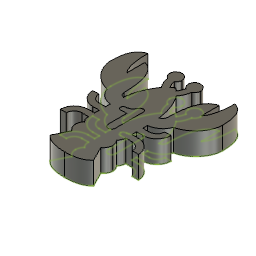
lobster-meeple-1 (Autodesk Fusion 360 design; units mm, degrees)
part number: 2026-09-20-14-42-37-938
Autodesk Fusion 360 part; units mm, degrees
sketch "Sketch4" plane through (0, 0, 0) normal (0, 0, 1) x (1, 0, 0)
  spline S0 degree 3 poles (20.1551, -11.6126) (23.0817, -10.9889) (25.2713, -8.149) (25.2713, -5.6734) knots 0 0 0 0 1 1 1 1
  spline S1 degree 2 poles (25.2713, -5.6734) (25.2713, -0.7748) (22.4721, -0.075) knots 0 0 0 1 1 1
  spline S2 degree 3 poles (22.4721, -0.075) (22.4721, -5.0901) (21.1273, -6.0667) (21.0725, -6.1398) knots 0 0 0 0 1 1 1 1
  line L0 (21.0725, -6.1398) -> (21.0725, -2.1744)
  spline S3 degree 3 poles (21.0725, -2.1744) (17.5735, -2.8742) (17.5735, -8.939) (17.5735, -10.3387) knots 0 0 0 0 1 1 1 1
  spline S4 degree 3 poles (17.5735, -10.3387) (17.5735, -10.8576) (17.1946, -11.2887) (16.6992, -11.3725) knots 0 0 0 0 1 1 1 1
  spline S5 degree 3 poles (16.6992, -11.3725) (16.295, -8.2827) (15.2588, -6.3478) (14.3388, -5.1927) knots 0 0 0 0 1 1 1 1
  spline S6 degree 3 poles (14.3388, -5.1927) (14.7426, -4.751) (15.2127, -3.9854) (15.3954, -2.7274) knots 0 0 0 0 1 1 1 1
  spline S7 degree 3 poles (15.3954, -2.7274) (15.8563, -2.4984) (16.1739, -2.0241) (16.1739, -1.4746) knots 0 0 0 0 1 1 1 1
  spline S8 degree 3 poles (16.1739, -1.4746) (16.1739, -0.7017) (15.5472, -0.075) (14.7743, -0.075) knots 0 0 0 0 1 1 1 1
  spline S9 degree 3 poles (14.7743, -0.075) (14.0013, -0.075) (13.3747, -0.7017) (13.3747, -1.4746) knots 0 0 0 0 1 1 1 1
  spline S10 degree 3 poles (13.3747, -1.4746) (13.3747, -1.9583) (13.6201, -2.3845) (13.9931, -2.636) knots 0 0 0 0 1 1 1 1
  spline S11 degree 3 poles (13.9931, -2.636) (13.859, -3.4351) (13.5844, -3.9119) (13.3647, -4.1785) knots 0 0 0 0 1 1 1 1
  spline S12 degree 2 poles (13.3647, -4.1785) (12.9526, -3.8299) (12.675, -3.6906) knots 0 0 0 1 1 1
  spline S13 degree 2 poles (12.675, -3.6906) (12.3973, -3.8299) (11.9853, -4.1785) knots 0 0 0 1 1 1
  spline S14 degree 3 poles (11.9853, -4.1785) (11.7655, -3.9119) (11.4909, -3.4351) (11.3568, -2.636) knots 0 0 0 0 1 1 1 1
  spline S15 degree 3 poles (11.3568, -2.636) (11.7298, -2.3845) (11.9753, -1.9582) (11.9753, -1.4746) knots 0 0 0 0 1 1 1 1
  spline S16 degree 3 poles (11.9753, -1.4746) (11.9753, -0.7017) (11.3486, -0.075) (10.5757, -0.075) knots 0 0 0 0 1 1 1 1
  spline S17 degree 3 poles (10.5757, -0.075) (9.8027, -0.075) (9.1761, -0.7017) (9.1761, -1.4746) knots 0 0 0 0 1 1 1 1
  spline S18 degree 3 poles (9.1761, -1.4746) (9.1761, -2.0242) (9.4936, -2.4984) (9.9545, -2.7274) knots 0 0 0 0 1 1 1 1
  spline S19 degree 3 poles (9.9545, -2.7274) (10.1372, -3.9854) (10.6074, -4.751) (11.0111, -5.1927) knots 0 0 0 0 1 1 1 1
  spline S20 degree 3 poles (11.0111, -5.1927) (10.0912, -6.3478) (9.055, -8.2827) (8.6508, -11.3725) knots 0 0 0 0 1 1 1 1
  spline S21 degree 3 poles (8.6508, -11.3725) (8.1553, -11.2887) (7.7765, -10.8576) (7.7765, -10.3387) knots 0 0 0 0 1 1 1 1
  spline S22 degree 3 poles (7.7765, -10.3387) (7.7765, -8.9391) (7.7765, -2.8742) (4.2775, -2.1744) knots 0 0 0 0 1 1 1 1
  line L1 (4.2775, -2.1744) -> (4.2775, -6.1398)
  spline S23 degree 3 poles (4.2775, -6.1398) (4.2226, -6.0667) (2.8779, -5.0901) (2.8779, -0.075) knots 0 0 0 0 1 1 1 1
  spline S24 degree 2 poles (2.8779, -0.075) (0.0787, -0.7748) (0.0787, -5.6734) knots 0 0 0 1 1 1
  spline S25 degree 3 poles (0.0787, -5.6734) (0.0787, -8.149) (2.2683, -10.989) (5.1949, -11.6126) knots 0 0 0 0 1 1 1 1
  spline S26 degree 3 poles (5.1949, -11.6126) (5.6849, -13.0051) (6.9538, -14.0331) (8.4764, -14.1709) knots 0 0 0 0 1 1 1 1
  spline S27 degree 3 poles (8.4764, -14.1709) (8.4764, -14.1765) (8.4763, -14.1819) (8.4763, -14.1875) knots 0 0 0 0 1 1 1 1
  line L2 (8.4763, -14.1875) -> (8.4763, -15.2372)
  line L3 (8.4763, -15.2372) -> (7.0067, -15.2372)
  spline S28 degree 3 poles (7.0067, -15.2372) (6.042, -15.2372) (5.2572, -14.4524) (5.2572, -13.4877) knots 0 0 0 0 1 1 1 1
  line L4 (5.2572, -13.4877) -> (3.8576, -13.4877)
  spline S29 degree 3 poles (3.8576, -13.4877) (3.8576, -15.2241) (5.2703, -16.6368) (7.0067, -16.6368) knots 0 0 0 0 1 1 1 1
  line L5 (7.0067, -16.6368) -> (8.4763, -16.6368)
  line L6 (8.4763, -16.6368) -> (8.4763, -17.6865)
  line L7 (8.4763, -17.6865) -> (7.0067, -17.6865)
  spline S30 degree 3 poles (7.0067, -17.6865) (5.2703, -17.6865) (3.8576, -19.0992) (3.8576, -20.8356) knots 0 0 0 0 1 1 1 1
  line L8 (3.8576, -20.8356) -> (5.2572, -20.8356)
  spline S31 degree 3 poles (5.2572, -20.8356) (5.2572, -19.8709) (6.042, -19.0861) (7.0067, -19.0861) knots 0 0 0 0 1 1 1 1
  line L9 (7.0067, -19.0861) -> (8.4763, -19.0861)
  spline S32 degree 3 poles (8.4763, -19.0861) (8.4763, -19.6526) (8.7011, -20.1663) (9.0659, -20.544) knots 0 0 0 0 1 1 1 1
  spline S33 degree 3 poles (9.0659, -20.544) (8.7011, -20.9216) (8.4763, -21.4353) (8.4763, -22.0018) knots 0 0 0 0 1 1 1 1
  spline S34 degree 3 poles (8.4763, -22.0018) (8.4763, -22.7303) (8.8474, -23.3719) (9.4109, -23.7484) knots 0 0 0 0 1 1 1 1
  line L10 (9.4109, -23.7484) -> (7.7764, -27.0171)
  spline S35 degree 2 poles (7.7764, -27.0171) (9.1209, -28.65) (12.675, -28.65) knots 0 0 0 1 1 1
  spline S36 degree 2 poles (12.675, -28.65) (16.229, -28.65) (17.5736, -27.0171) knots 0 0 0 1 1 1
  line L11 (17.5736, -27.0171) -> (15.9393, -23.7485)
  spline S37 degree 3 poles (15.9393, -23.7485) (16.5027, -23.372) (16.8738, -22.7304) (16.8738, -22.0019) knots 0 0 0 0 1 1 1 1
  spline S38 degree 3 poles (16.8738, -22.0019) (16.8738, -21.4354) (16.6489, -20.9217) (16.2842, -20.544) knots 0 0 0 0 1 1 1 1
  spline S39 degree 3 poles (16.2842, -20.544) (16.6489, -20.1664) (16.8738, -19.6526) (16.8738, -19.0861) knots 0 0 0 0 1 1 1 1
  line L12 (16.8738, -19.0861) -> (18.3433, -19.0861)
  spline S40 degree 3 poles (18.3433, -19.0861) (19.308, -19.0861) (20.0928, -19.871) (20.0928, -20.8356) knots 0 0 0 0 1 1 1 1
  line L13 (20.0928, -20.8356) -> (21.4924, -20.8356)
  spline S41 degree 3 poles (21.4924, -20.8356) (21.4924, -19.0992) (20.0798, -17.6866) (18.3433, -17.6866) knots 0 0 0 0 1 1 1 1
  line L14 (18.3433, -17.6866) -> (16.8738, -17.6866)
  line L15 (16.8738, -17.6866) -> (16.8738, -16.6369)
  line L16 (16.8738, -16.6369) -> (18.3433, -16.6369)
  spline S42 degree 3 poles (18.3433, -16.6369) (20.0798, -16.6369) (21.4924, -15.2242) (21.4924, -13.4878) knots 0 0 0 0 1 1 1 1
  line L17 (21.4924, -13.4878) -> (20.0928, -13.4878)
  spline S43 degree 3 poles (20.0928, -13.4878) (20.0928, -14.4524) (19.308, -15.2373) (18.3433, -15.2373) knots 0 0 0 0 1 1 1 1
  line L18 (18.3433, -15.2373) -> (16.8738, -15.2373)
  line L19 (16.8738, -15.2373) -> (16.8738, -14.1876)
  spline S44 degree 3 poles (16.8738, -14.1876) (16.8738, -14.182) (16.8736, -14.1765) (16.8736, -14.171) knots 0 0 0 0 1 1 1 1
  spline S45 degree 3 poles (16.8736, -14.171) (18.3963, -14.0331) (19.6651, -13.0051) (20.1551, -11.6126) knots 0 0 0 0 1 1 1 1
  spline S46 degree 3 poles (12.1852, -18.1975) (12.1852, -18.7496) (12.3976, -19.1317) (12.9921, -19.1317) knots 0 0 0 0 1 1 1 1
  spline S47 degree 3 poles (12.9921, -19.1317) (13.5866, -19.1317) (13.7989, -18.7496) (13.7989, -18.1975) knots 0 0 0 0 1 1 1 1
  line L20 (13.7989, -18.1975) -> (13.7989, -12.1675)
  spline S48 degree 3 poles (13.7989, -12.1675) (13.7989, -11.5942) (13.5229, -11.4456) (13.1832, -11.4456) knots 0 0 0 0 1 1 1 1
  spline S49 degree 3 poles (13.1832, -11.4456) (12.2808, -11.4456) (12.6099, -12.6558) (11.4315, -12.9106) knots 0 0 0 0 1 1 1 1
  line L21 (11.4315, -12.9106) -> (11.0387, -12.9956)
  spline S50 degree 3 poles (11.0387, -12.9956) (10.4866, -13.1017) (10.2743, -13.2079) (10.2743, -13.6007) knots 0 0 0 0 1 1 1 1
  spline S51 degree 3 poles (10.2743, -13.6007) (10.2743, -14.0359) (10.4654, -14.1633) (10.8158, -14.1633) knots 0 0 0 0 1 1 1 1
  line L22 (10.8158, -14.1633) -> (12.1852, -14.1633)
  line L23 (12.1852, -14.1633) -> (12.1852, -18.1975)
extrude "Extrude1" add sketch "Sketch4" along normal blind 5 makes body 1
extrude "Extrude2" add sketch "Sketch4" along normal blind 4.5 contours S46 S47 L20 S48 S49 L21 S50 S51 L22 L23 bodies 1
extrude "Extrude3" add 1 faces at (13.261, -14.8428, 4.5) along direction (0, 0, 1) blind 0.5 separate body on bodies 1 makes body 2
